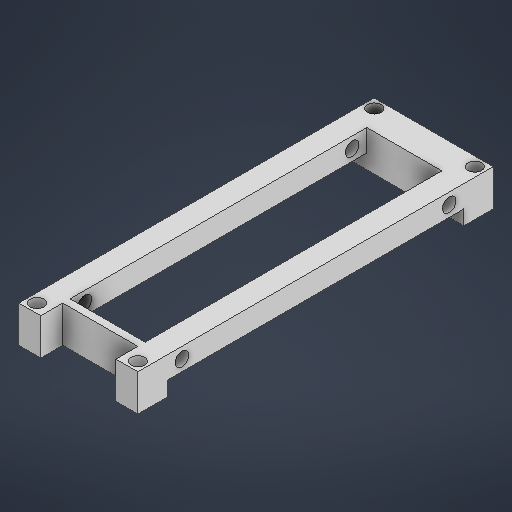
# Autodesk Inventor part: V1 screen holder
Saved by Autodesk Inventor 2026.2 (Build 302298000, 298)
## iProperties
Created: 2026-08-02
Part Number: V1 screen holder
Material: Generic
Document SubType Name: Modeling
Designer: Graeme
Density: 1 g/cm^3
Appearance: Default
Author: Graeme
## iProperties of the stored document V1 screen holder_3DPrint.ipt
Created: 2026-08-02
Part Number: V1 screen holder_3DPrint
Material: Generic
Document SubType Name: Modeling
Designer: Graeme
Density: 1 g/cm^3
Appearance: Default
Author: Graeme
Autodesk Inventor part; units mm, degrees
ref_plane "YZ Plane" through (0, 0, 0) normal (1, 0, 0) x (0, 1, 0)
ref_plane "XZ Plane" through (0, 0, 0) normal (0, 1, 0) x (-1, 0, 0)
ref_plane "XY Plane" through (0, 0, 0) normal (0, 0, 1) x (1, 0, 0)
sketch "Sketch1" plane through (0, 0, 0) normal (0, 1, 0) x (-1, 0, 0)
  line L0 (16.25, 48.5) -> (-16.25, 48.5)
  line L1 (-16.25, 48.5) -> (-16.25, -48.5)
  line L2 (-16.25, -48.5) -> (16.25, -48.5)
  line L3 (16.25, -48.5) -> (16.25, 48.5)
  line L4 (16.25, 48.5) -> (-16.25, -48.5) construction
  line L5 (-16.25, 48.5) -> (16.25, -48.5) construction
  line L6 (16.25, 48.5) -> (16.25, 40.5)
  line L7 (16.25, -48.5) -> (16.25, -40.5)
  line L8 (16.25, 40.5) -> (-16.25, 40.5)
  line L9 (16.25, -40.5) -> (-16.25, -40.5)
  line L10 (0, 48.5) -> (0, 42.5)
  line L11 (-16.25, 48.5) -> (-10.25, 48.5)
  line L12 (-10.25, 48.5) -> (-10.25, 42.5)
  line L13 (-10.25, 42.5) -> (-16.25, 42.5)
  line L14 (-16.25, 42.5) -> (-16.25, 48.5)
  line L15 (16.25, 48.5) -> (10.25, 48.5)
  line L16 (10.25, 48.5) -> (10.25, 42.5)
  line L17 (10.25, 42.5) -> (16.25, 42.5)
  line L18 (16.25, 42.5) -> (16.25, 48.5)
  line L19 (10.25, 42.5) -> (-10.25, 42.5)
  point P0 (0, 0)
  dimension "d0" = 32.5
  dimension "d1" = 97
  dimension "d4" = 6
  dimension "d5" = 6
  dimension "d6" = 6
  dimension "d7" = 6
  dimension "d8" = 6
  constraints: 40 end point, 6 parallel, 5 perpendicular, 4 point on line, 3 horizontal, 3 midpoint, 1 vertical
  measures "d0" distance of L2.end L1.end
  measures "d1" distance of L1.end L0.end
  measures "d4" distance of L10.start L10.end
  measures "d5" distance of L12.end L13.end
  measures "d6" distance of L11.end L12.end
  measures "d7" distance of L17.end L16.end
  measures "d8" distance of L16.end L15.end
extrude "Extrusion1" add sketch "Sketch1" along normal blind 10 contours L3 L17 L16 L0 | L3 L8 L1 L13 L19 L17 | L12 L13 L1 L0 | L3 L2 L1 L9
sketch "Sketch2" plane through (-16.25, 0, -40.5) normal (0, 0, 1) x (1, 0, 0)
  line L0 (0, 10) -> (32.5, 10) projected
  line L1 (32.5, 10) -> (26.5, 10)
  line L2 (26.5, 10) -> (26.5, 4)
  line L3 (26.5, 4) -> (32.5, 4)
  line L4 (32.5, 4) -> (32.5, 10)
  line L5 (0, 0) -> (0, 10) projected
  line L6 (0, 10) -> (6, 10)
  line L7 (6, 10) -> (6, 4)
  line L8 (6, 4) -> (0, 4)
  line L9 (0, 4) -> (0, 10)
  point P0 (16.25, 0)
  dimension "d11" = 6
  dimension "d12" = 6
  dimension "d15" = 6
  dimension "d16" = 6
  constraints: 16 end point, 4 parallel, 2 horizontal, 2 perpendicular
  measures "d11" distance of L3.end L2.end
  measures "d12" distance of L2.end L1.end
  measures "d15" distance of L7.end L8.end
  measures "d16" distance of L6.end L7.end
extrude "Extrusion2" add sketch "Sketch2" along normal up to surface (81 mm away)
sketch "Sketch3" plane through (-16.25, 0, -48.5) normal (-1, 0, 0) x (0, 0, 1)
  circle A0 centre (85, 7) radius 1.85
  circle A1 centre (12, 7) radius 1.85
  line L0 (8, 4) -> (89, 4) projected
  line L1 (97, 0) -> (97, 10) projected
  line L2 (0, 0) -> (0, 10) projected
  point P0 (48.5, 0)
  dimension "d17" = 3.7
  dimension "d18" = 3.7
  dimension "d19" = 3
  dimension "d20" = 3
  dimension "d21" = 12
  dimension "d22" = 12
  constraints: 2 centre point
  measures "d17" diameter of A0
  measures "d18" diameter of A1
  measures "d19" distance from line of L0 A0.centre
  measures "d20" distance from line of L0 A1.centre
  measures "d21" distance from line of A0.centre L1
  measures "d22" distance from line of L2 A1.centre
extrude "Extrusion3" cut sketch "Sketch3" against normal up to surface (32.5 mm away)
sketch "Sketch4" plane through (0, 0, 0) normal (0, -1, 0) x (1, 0, 0)
  circle A0 centre (13.75, 46) radius 1.85
  circle A1 centre (13.75, -46) radius 1.85
  circle A2 centre (-13.75, -46) radius 1.85
  circle A3 centre (-13.75, 46) radius 1.85
  line L0 (10.25, 48.5) -> (16.25, 48.5) projected
  line L1 (16.25, 48.5) -> (16.25, 40.5) projected
  line L2 (-16.25, 48.5) -> (-10.25, 48.5) projected
  line L3 (-16.25, 40.5) -> (-16.25, 48.5) projected
  line L4 (16.25, -40.5) -> (16.25, -48.5) projected
  line L5 (16.25, -48.5) -> (-16.25, -48.5) projected
  line L6 (-16.25, -48.5) -> (-16.25, -40.5) projected
  point P0 (0, 0)
  point P1 (16.25, 44.5)
  dimension "d25" = 3.7
  dimension "d26" = 3.7
  dimension "d27" = 3.7
  dimension "d28" = 3.7
  dimension "d29" = 2.5
  dimension "d30" = 2.5
  dimension "d31" = 2.5
  dimension "d32" = 2.5
  dimension "d33" = 2.5
  dimension "d34" = 2.5
  dimension "d35" = 2.5
  dimension "d36" = 2.5
  constraints: 4 centre point, 1 midpoint
  measures "d25" diameter of A0
  measures "d26" diameter of A1
  measures "d27" diameter of A2
  measures "d28" diameter of A3
  measures "d29" distance from line of A0.centre L0
  measures "d30" horizontal distance of point (16.25, 44.5) A0.centre
  measures "d31" distance from line of L2 A3.centre
  measures "d32" distance from line of L3 A3.centre
  measures "d33" distance from line of L4 A1.centre
  measures "d34" distance from line of L5 A1.centre
  measures "d35" distance from line of L5 A2.centre
  measures "d36" distance from line of L6 A2.centre
extrude "Extrusion4" cut sketch "Sketch4" against normal blind 10
equation "\"d18\" = d17"
equation "\"d20\" = d19"
equation "\"d30\" = d29"
equation "\"d31\" = d29"
equation "\"d32\" = d29"
equation "\"d33\" = d29"
equation "\"d34\" = d29"
equation "\"d35\" = d29"
equation "\"d36\" = d29"
body "Solid1"
